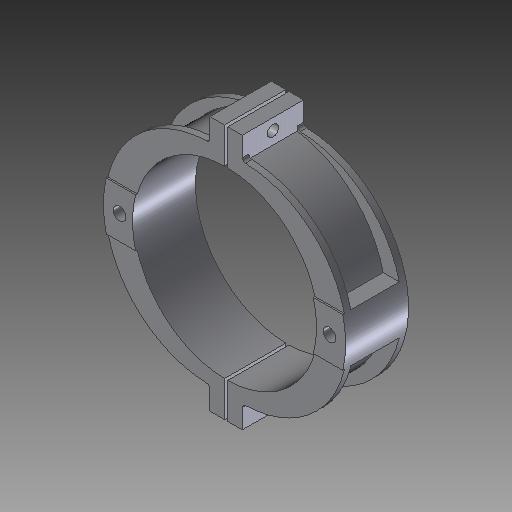
# Autodesk Inventor part: 3211_Bed Rail Clamp
Saved by Autodesk Inventor 2020 (Build 240168000, 168)
## iProperties
Created: 2019-06-17
Part Number: 3211_Bed Rail Clamp
Material: Acetal Resin, White
Document SubType Name: Sheet Metal
Designer: MPI
Density: 1.425 g/cm^3
Sheet Metal Rule: Default_mm
Appearance: Smooth - White
Mass: 241.345 g
Surface Area: 545.86 cm^2
Volume: 169.365 cm^3
Author: MPI
Autodesk Inventor part; units mm, degrees
ref_plane "YZ Plane" through (0, 0, 0) normal (1, 0, 0) x (0, 1, 0)
ref_plane "XZ Plane" through (0, 0, 0) normal (0, 1, 0) x (-1, 0, 0)
ref_plane "XY Plane" through (0, 0, 0) normal (0, 0, 1) x (1, 0, 0)
sketch "Sketch1" plane through (0, 0, 0) normal (0, 0, 1) x (1, 0, 0)
  arc A0 (-10, 65) -> (-10, -65) centre (-10, 0) ccw
  arc A1 (10, -65) -> (10, 65) centre (10, 0) ccw
  line L0 (-10, 65) -> (-10, 79)
  line L1 (10, -79) -> (10, -65)
  line L2 (10, 65) -> (10, 79)
  line L3 (-10, -79) -> (-10, -65)
  line L4 (1, -119) -> (-1, -119)
  line L5 (-1, -79) -> (-1, -56.9912)
  line L6 (-1, 56.9912) -> (-1, 79)
  line L7 (1, 79) -> (1, 56.9912)
  line L8 (1, -56.9912) -> (1, -79)
  line L9 (-10, -79) -> (-1, -79)
  line L10 (1, -79) -> (10, -79)
  line L11 (-10, 79) -> (-1, 79)
  line L12 (1, 79) -> (10, 79)
  arc A2 (1, -56.9912) -> (1, 56.9912) centre (0, 0) ccw
  arc A3 (-1, 56.9912) -> (-1, -56.9912) centre (0, 0) ccw
  circle A4 centre (0, 0) radius 65 construction
  dimension "d11" = 14
  dimension "d16" = 130
  dimension "d70" = 65
  dimension "d71" = 57
  dimension "d72" = 9
  constraints: 26 end point, 8 point on circle, 6 parallel, 5 centre point, 4 horizontal, 4 vertical, 2 coincident
  measures "d11" distance of L2.start L2.end
  measures "d16" diameter of A4
  measures "d70" radius of A0
  measures "d71" radius of A3
  measures "d72" distance of L7.start L2.end
extrude "Extrusion1" add sketch "Sketch1" along normal blind 4
sketch "Sketch2" plane through (0, 0, 4) normal (0, 0, 1) x (1, 0, 0)
  line L0 (0, 0) -> (-10, 0)
  line L1 (0, 0) -> (10, 0)
  arc A0 (73.2456, -15) -> (73.2456, 15) centre (10, 0) ccw
  arc A1 (-73.2456, 15) -> (-73.2456, -15) centre (-10, 0) ccw
  arc A2 (-54.9909, 15) -> (-54.9909, -15) centre (0, 0) ccw
  arc A3 (54.9909, -15) -> (54.9909, 15) centre (0, 0) ccw
  line L2 (-73.2456, 15) -> (-63.2456, 15)
  line L3 (63.2456, 15) -> (73.2456, 15)
  line L4 (73.2456, -15) -> (63.2456, -15)
  line L5 (-63.2456, -15) -> (-73.2456, -15)
  line L6 (10, 79) -> (10, 64.2262)
  line L7 (-10, 64.2262) -> (-10, 79)
  line L8 (10, 79) -> (1, 79) projected
  line L9 (-10, 79) -> (-10, 65) projected
  line L10 (10, 65) -> (10, 79) projected
  line L11 (-1, 56.9912) -> (-1, 79) projected
  line L12 (-1, 79) -> (-1, 65)
  line L13 (1, 56.9912) -> (1, 79) projected
  line L14 (1, 79) -> (1, 65)
  line L15 (-10, 79) -> (-1, 79)
  line L16 (1, 79) -> (10, 79)
  line L17 (10, -64.2262) -> (10, -79)
  line L18 (-10, -79) -> (-10, -64.2262)
  line L19 (-10, -65) -> (-10, -79) projected
  line L20 (10, -79) -> (10, -65) projected
  line L21 (1, -79) -> (10, -79) projected
  line L22 (-1, -79) -> (-1, -56.9912) projected
  line L23 (-1, -65) -> (-1, -79)
  line L24 (1, -79) -> (1, -56.9912) projected
  line L25 (1, -65) -> (1, -79)
  line L26 (10, -79) -> (1, -79)
  line L27 (-1, -79) -> (-10, -79)
  arc A4 (-63.2456, -15) -> (-10, -64.2262) centre (0, 0) ccw
  arc A5 (10, -64.2262) -> (63.2456, -15) centre (0, 0) ccw
  arc A6 (63.2456, 15) -> (10, 64.2262) centre (0, 0) ccw
  arc A7 (-10, 64.2262) -> (-63.2456, 15) centre (0, 0) ccw
  arc A8 (1, -56.9912) -> (1, 56.9912) centre (0, 0) ccw
  arc A9 (-1, 56.9912) -> (-1, -56.9912) centre (0, 0) ccw
  line L28 (-1, 64.9923) -> (-1, 56.9912)
  line L29 (1, 56.9912) -> (1, 64.9923)
  line L30 (-1, -56.9912) -> (-1, -64.9923)
  line L31 (1, -56.9912) -> (1, -64.9923)
  line L32 (1, -56.9912) -> (1, -79) projected
  point P0 (-10, 65)
  dimension "d17" = 10
  dimension "d19" = 10
  dimension "d23" = 15
  dimension "d24" = 15
  dimension "d73" = 14
  dimension "d74" = 14
  constraints: 48 end point, 20 point on circle, 14 collinear, 10 centre point, 7 point on line, 6 horizontal, 6 parallel, 5 coincident, 2 perpendicular
  measures "d17" distance of L0.start L0.end
  measures "d19" distance of L0.start L1.end
  measures "d23" distance from line of point (0, 0) L2
  measures "d24" distance from line of point (0, 0) L5
  measures "d73" distance of L25.start L21.start
  measures "d74" distance of L8.end L14.end
extrude "Extrusion2" add sketch "Sketch2" along normal blind 34
sketch "Sketch3" plane through (0, 0, 38) normal (0, 0, 1) x (1, 0, 0)
  line L0 (0, 0) -> (-10, 0)
  line L1 (0, 0) -> (10, 0)
  line L2 (-10, 79) -> (-1, 79)
  line L3 (-1, 79) -> (-1, 56.9912)
  line L4 (-1, 79) -> (-10, 79) projected
  line L5 (-1, 56.9912) -> (-1, 79) projected
  line L6 (1, 79) -> (10, 79)
  line L7 (10, 79) -> (10, 65)
  line L8 (10, 62) -> (9.5192, 62)
  line L9 (1, 56.9912) -> (1, 79)
  line L10 (10, 79) -> (1, 79) projected
  line L11 (1, 79) -> (1, 56.9912) projected
  line L12 (-1, -56.9912) -> (-1, -79)
  line L13 (-1, -79) -> (-10, -79)
  line L14 (-10, -79) -> (-10, -65)
  line L15 (-1, -79) -> (-1, -56.9912) projected
  line L16 (-10, -79) -> (-1, -79) projected
  arc A0 (-10, 65) -> (-10, -65) centre (-10, 0) ccw
  line L17 (10, -65) -> (10, -79)
  line L18 (10, -79) -> (1, -79)
  line L19 (10, -79) -> (10, -64.2262) projected
  line L20 (1, -79) -> (10, -79) projected
  arc A1 (10, -65) -> (10, 65) centre (10, 0) ccw
  arc A2 (-1, 56.9912) -> (-1, -56.9912) centre (0, 0) ccw
  arc A3 (1, -56.9912) -> (1, 56.9912) centre (0, 0) ccw
  line L21 (1, -56.9912) -> (1, -79)
  line L22 (-10, 79) -> (-10, 65) projected
  line L23 (-10, 79) -> (-10, 65)
  point P0 (-1, 65)
  point P1 (1, 65)
  point P2 (-1, -65)
  dimension "d31" = 10
  dimension "d32" = 10
  constraints: 30 end point, 11 point on circle, 9 collinear, 4 centre point, 4 horizontal, 3 coincident, 3 parallel, 2 perpendicular, 1 point on line, 1 vertical
  measures "d31" distance of L0.start L0.end
  measures "d32" distance of L0.start L1.end
extrude "Extrusion3" add sketch "Sketch3" against normal blind 4
fillet "Fillet1" radius 2 8 edges at (-10, 65, 2) (10, 65, 2) (-10, -65, 2) (10, -65, 2) (10, 65, 36) (10, -65, 36) (-10, -65, 36) (-10, 65, 36)
sketch "Sketch5" plane through (0, 0, 38) normal (0, 0, 1) x (1, 0, 0)
  arc A0 (-73.2456, 15) -> (-73.2456, -15) centre (-10, 0) ccw
  line L0 (-73.2456, 15) -> (-54.9909, 15)
  line L1 (54.9909, 15) -> (73.2456, 15)
  line L2 (73.2456, -15) -> (54.9909, -15)
  line L3 (-54.9909, -15) -> (-73.2456, -15)
  arc A1 (-54.9909, 15) -> (-54.9909, -15) centre (0, 0) ccw
  arc A2 (54.9909, -15) -> (54.9909, 15) centre (0, 0) ccw
  arc A3 (73.2456, -15) -> (73.2456, 15) centre (10, 0) ccw
  constraints: 8 end point, 8 point on circle, 4 centre point, 4 parallel, 2 horizontal, 1 coincident
extrude "Extrusion5" add sketch "Sketch5" along normal blind 1
sketch "Sketch6" plane through (-10, 65, 38) normal (-1, 0, 0) x (0, 0, 1)
  circle A0 centre (-19, 7) radius 3.5
  line L0 (-38, 14) -> (0, 14) projected
  line L1 (-38, 14) -> (-38, 1.9701) projected
  circle A1 centre (-19, -137) radius 3.5
  line L2 (-38, -131.9701) -> (-38, -144) projected
  line L3 (-38, -144) -> (0, -144) projected
  point P0 (-38, -65)
  dimension "d56" = 7
  dimension "d57" = 7
  dimension "d58" = 19
  dimension "d59" = 7
  dimension "d75" = 19
  dimension "d76" = 7
  constraints: 2 centre point
  measures "d56" diameter of A0
  measures "d57" distance from line of A0.centre L0
  measures "d58" distance from line of A0.centre L1
  measures "d59" diameter of A1
  measures "d75" distance from line of A1.centre L2
  measures "d76" distance from line of A1.centre L3
extrude "Extrusion6" cut sketch "Sketch6" against normal through all
sketch "Sketch7" plane through (0, 0, 39) normal (0, 0, 1) x (1, 0, 0)
  circle A0 centre (-65, 0) radius 4
  circle A1 centre (65, 0) radius 4
  point P0 (0, 0)
  dimension "d65" = 8
  dimension "d66" = 8
  constraints: 2 centre point
  measures "d65" diameter of A0
  measures "d66" diameter of A1
extrude "Extrusion7" cut sketch "Sketch7" against normal through all
equation "\"BendRadius\" = Thickness"
equation "\"BendReliefWidth\" = Thickness"
equation "\"BendReliefDepth\" = 0.5 * Thickness"
equation "\"CornerReliefSize\" = 4 * Thickness"
equation "\"MinimumRemnant\" = 2 * Thickness"
equation "\"TransitionRadius\" = BendRadius"
equation "\"JacobiRadiusSize\" = BendRadius"
equation "\"GapSize\" = Thickness"
equation "\"Thickness\" = 0.5"
body "Solid1"
